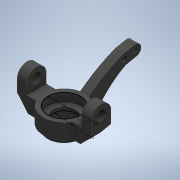
# Autodesk Inventor part: RCT-P006_steering_knuckle
Saved by Autodesk Inventor 2020 (Build 240168000, 168)
## iProperties
Created: 2018-12-11
Part Number: RCT-P006_steering_knuckle
Material: Generic
Document SubType Name: Modeling
Designer: Ehecatl Eli
Density: 1 g/cm^3
Appearance: Generic
Author: Ehecatl Eli
Autodesk Inventor part; units mm, degrees
ref_plane "YZ Plane" through (0, 0, 0) normal (1, 0, 0) x (0, 1, 0)
ref_plane "XZ Plane" through (0, 0, 0) normal (0, 1, 0) x (-1, 0, 0)
ref_plane "XY Plane" through (0, 0, 0) normal (0, 0, 1) x (1, 0, 0)
sketch "Sketch1" plane through (0, 0, 0) normal (0, 0, 1) x (1, 0, 0)
  line L0 (17, 4.5) -> (17, -4.5)
  line L1 (-17, -4.5) -> (-17, 4.5)
  arc A0 (-8.3666, -4.5) -> (8.3666, -4.5) centre (0, 0) ccw
  arc A1 (8.3666, 4.5) -> (-8.3666, 4.5) centre (0, 0) ccw
  line L2 (-17, 4.5) -> (-8.3666, 4.5)
  line L3 (8.3666, 4.5) -> (17, 4.5)
  line L4 (17, -4.5) -> (8.3666, -4.5)
  line L5 (-8.3666, -4.5) -> (-17, -4.5)
  line L6 (-17, 4.5) -> (17, -4.5) construction
  line L7 (-17, -4.5) -> (17, 4.5) construction
  point P0 (0, 0)
  point P1 (0, 0)
  dimension "d0" = 9
  dimension "d1" = 34
  dimension "d2" = 9.5
  dimension "d3" = 9
  dimension "d4" = 9.5
  dimension "d12" = 4.5
  constraints: 16 end point, 5 parallel, 4 point on circle, 2 centre point, 2 coincident, 2 horizontal, 2 midpoint, 2 perpendicular
  measures "d0" distance of L1.start L1.end
  measures "d1" distance between parallel lines of L0 L1
  measures "d2" radius of A1
  measures "d3" distance of L0.start L0.end
  measures "d4" radius of A0
  measures "d12" distance from line of point (0, 0) L5
extrude "Extrusion1" add sketch "Sketch1" along normal blind 7
sketch "Sketch2" plane through (17, -4.5, 0) normal (1, 0, 0) x (0, 0, -1)
  arc A0 (-11.5, 9) -> (-11.5, 0) centre (-11.5, 4.5) ccw
  circle A1 centre (-11.5, 4.5) radius 2.25
  line L0 (-7, 9) -> (-11.5, 9)
  line L1 (-11.5, 0) -> (-7, 0)
  line L2 (-7, 0) -> (-7, 9)
  point P0 (0, 4.5)
  point P1 (-7, 0)
  dimension "d7" = 9
  dimension "d8" = 4.5
  dimension "d9" = 9
  constraints: 6 end point, 2 centre point, 2 coincident, 2 horizontal, 2 point on circle, 2 tangent, 1 parallel, 1 vertical
  measures "d7" diameter of A0
  measures "d8" diameter of A1
extrude "Extrusion2" add sketch "Sketch2" against normal blind 4.3
extrude "Extrusion3" add sketch "Sketch2" along normal blind 4.3 from surface at -34
sketch "Sketch3" plane through (-17, -4.5, 0) normal (0, -1, 0) x (1, 0, 0)
  line L0 (0, 6) -> (0, 0)
  line L1 (0, 0) -> (5, 0)
  line L2 (5, 0) -> (0, 6)
  line L3 (29, 0) -> (34, 0)
  line L4 (34, 0) -> (34, 6)
  line L5 (34, 6) -> (29, 0)
  point P0 (17, 0)
  dimension "d15" = 6
  dimension "d16" = 5
  dimension "d17" = 6
  dimension "d18" = 5
  constraints: 12 end point, 2 coincident, 2 perpendicular, 1 horizontal, 1 vertical
  measures "d15" distance of L0.start L0.end
  measures "d16" distance of L0.end L1.end
  measures "d17" distance of L3.end L4.end
  measures "d18" distance of L3.start L3.end
extrude "Extrusion4" cut sketch "Sketch3" against normal up to next
sketch "Sketch4" plane through (0, 0, 0) normal (0, 0, -1) x (-1, 0, 0)
  circle A0 centre (0, 0) radius 7.5
  dimension "d21" = 15
  constraints: 1 centre point, 1 coincident
  measures "d21" diameter of A0
extrude "Extrusion5" add sketch "Sketch4" along normal blind 2.5
sketch "Sketch5" plane through (0, 0, 7) normal (0, 0, 1) x (1, 0, 0)
  circle A0 centre (0, 0) radius 7.5
  dimension "d24" = 15
  constraints: 1 centre point, 1 coincident
  measures "d24" diameter of A0
extrude "Extrusion6" cut sketch "Sketch5" against normal blind 4
sketch "Sketch6" plane through (0, 0, -2.5) normal (0, 0, -1) x (-1, 0, 0)
  circle A0 centre (0, 0) radius 5.5
  dimension "d27" = 11
  constraints: 1 centre point, 1 coincident
  measures "d27" diameter of A0
extrude "Extrusion7" cut sketch "Sketch6" against normal blind 4
sketch "Sketch7" plane through (0, 0, 1.5) normal (0, 0, -1) x (-1, 0, 0)
  circle A0 centre (0, 0) radius 5
  dimension "d30" = 10
  constraints: 1 centre point, 1 coincident
  measures "d30" diameter of A0
extrude "Extrusion8" cut sketch "Sketch7" against normal up to next
sketch "Sketch9" plane through (0, 0, 0) normal (1, 0, 0) x (0, 1, 0)
  line L0 (-9.5504, 0) -> (57.3026, 0) projected
  line L1 (0, -37.6235) -> (0, 29.8791) projected
  line L2 (9.5, 0) -> (4.5, 0) projected
  line L3 (9.5, 7) -> (4.5, 7) projected
  circle A0 centre (30.75, 14.5) radius 1.25
  circle A1 centre (25.75, 13.5) radius 1.25
  line L4 (8.5, 7) -> (9.5, 7)
  line L5 (13.5, 7) -> (13.5, 0) construction
  line L6 (12.4966, 0) -> (8.5, 0)
  line L7 (8.5, 0) -> (8.5, 7)
  line L8 (25.75, 13.5) -> (30.75, 14.5) construction
  line L9 (26.2403, 11.0485) -> (31.2403, 12.0485)
  line L10 (30.2597, 16.9515) -> (25.2597, 15.9515)
  arc A2 (25.2597, 15.9515) -> (26.2403, 11.0485) centre (25.75, 13.5) ccw construction
  arc A3 (31.2403, 12.0485) -> (30.2597, 16.9515) centre (30.75, 14.5) ccw
  arc A4 (25.2597, 15.9515) -> (9.5, 7) centre (49.2826, -44.6916) ccw
  arc A5 (26.2403, 11.0485) -> (14.0842, 0.7836) centre (43.5805, -21.8166) ccw
  arc A6 (12.4966, 0) -> (14.0842, 0.7836) centre (12.4966, 2) ccw
  point P0 (0, 0)
  point P1 (28.25, 14)
  dimension "d133" = 2.5
  dimension "d134" = 30.75
  dimension "d135" = 14.5
  dimension "d136" = 2.5
  dimension "d137" = 13.5
  dimension "d138" = 25.75
  dimension "d139" = 7
  dimension "d140" = 5
  dimension "d141" = 8.5
  dimension "d142" = 5
  dimension "d143" = 65.2279
  dimension "d144" = 37.1592
  dimension "d145" = 2
  constraints: 16 end point, 12 point on circle, 7 centre point, 6 tangent, 3 parallel, 1 collinear, 1 horizontal, 1 midpoint, 1 perpendicular, 1 point on line
  measures "d133" diameter of A0
  measures "d134" distance from line of L1 L8.end
  measures "d135" distance from line of L0 L8.end
  measures "d136" diameter of A1
  measures "d137" distance from line of L0 L8.start
  measures "d138" distance from line of L1 L8.start
  measures "d139" distance of L5.start L5.end
  measures "d140" distance of L4.start L5.start
  measures "d141" distance between parallel lines of L1 L7
  measures "d142" diameter of A3
  measures "d143" radius of A4
  measures "d144" radius of A5
  measures "d145" radius of A6
extrude "Extrusion22" add sketch "Sketch9" along normal mid plane 4
body "Solid1"
